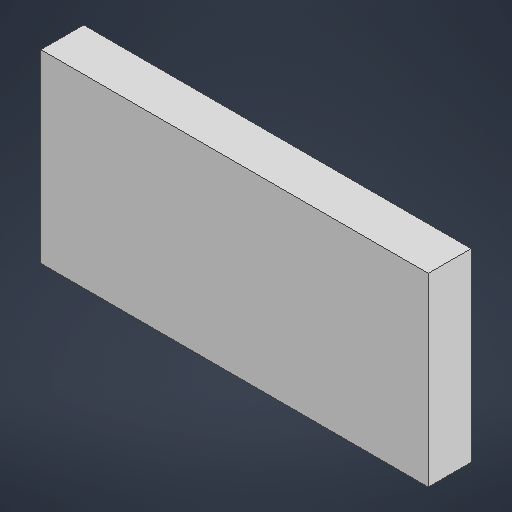
# Autodesk Inventor part: Battery
Saved by Autodesk Inventor 2026.1 (Build 301233020, 233B)
## iProperties
Created: 2025-12-01
Part Number: Battery
Material: Generic
Document SubType Name: Modeling
Designer: osama
Density: 1 g/cm^3
Appearance: Default
Author: osama
Autodesk Inventor part; units mm, degrees
ref_plane "YZ Plane" through (0, 0, 0) normal (1, 0, 0) x (0, 1, 0)
ref_plane "XZ Plane" through (0, 0, 0) normal (0, 1, 0) x (-1, 0, 0)
ref_plane "XY Plane" through (0, 0, 0) normal (0, 0, 1) x (1, 0, 0)
sketch "Sketch1" plane through (0, 0, 0) normal (0, 0, 1) x (1, 0, 0)
  line L0 (-73.25, -35) -> (73.25, -35)
  line L1 (73.25, -35) -> (73.25, 35)
  line L2 (73.25, 35) -> (-73.25, 35)
  line L3 (-73.25, 35) -> (-73.25, -35)
  line L4 (-73.25, -35) -> (73.25, 35) construction
  line L5 (73.25, -35) -> (-73.25, 35) construction
  point P0 (0, 0)
  dimension "d0" = 146.5
  dimension "d1" = 70
  constraints: 12 end point, 2 midpoint, 2 parallel, 1 horizontal, 1 perpendicular
  measures "d0" distance of L2.end L1.end
  measures "d1" distance of L1.end L0.end
extrude "Extrusion1" add sketch "Sketch1" along normal blind 16.2
body "Solid1"
